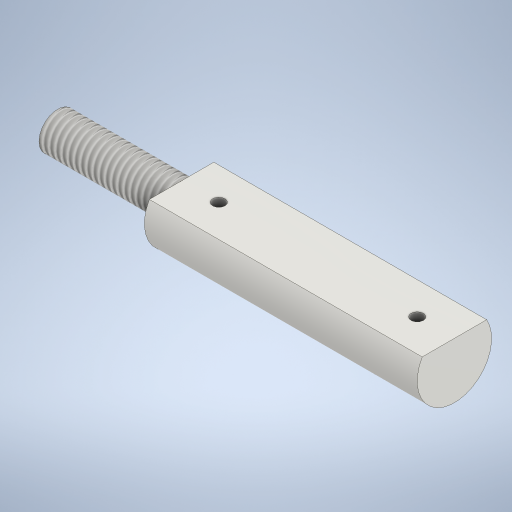
# Autodesk Inventor part: centre shaft
Saved by Autodesk Inventor 2023 (Build 270158000, 158)
## iProperties
CustomPartVersion: 1
Created: 2023-05-29
Part Number: centre shaft
Material: Steel
Document SubType Name: Modeling
Designer: Ronan
Density: 1 g/cm^3
Appearance: Steel
Length: 18,000 mm
Author: Ronan
Autodesk Inventor part; units mm, degrees
ref_plane "Start Plane" through (0, 0, 0) normal (1, 0, 0) x (0, 1, 0)
ref_plane "XZ Plane" through (0, 0, 0) normal (0, 1, 0) x (-1, 0, 0)
ref_plane "XY Plane" through (0, 0, 0) normal (0, 0, 1) x (1, 0, 0)
sketch "Sketch4" plane through (0, 0, 0) normal (1, 0, 0) x (0, 1, 0)
  circle A0 centre (0, 0) radius 3
  dimension "d11" = 6
  constraints: 1 centre point, 1 coincident
  measures "d11" diameter of A0
extrude "Extrusion2" add sketch "Sketch4" along normal blind 22
sketch "Sketch5" plane through (22, 0, 0) normal (1, 0, 0) x (0, 0, -1)
  circle A0 centre (0, 0) radius 3 projected
  line L0 (-2.5981, 1.5) -> (2.5981, 1.5)
  circle A1 centre (0, 0) radius 3
  dimension "d14" = 1.5
  constraints: 2 end point, 2 point on circle, 1 centre point, 1 coincident, 1 concentric, 1 horizontal
  measures "d14" distance from line of point (0, 0) L0
extrude "Extrusion3" cut sketch "Sketch5" against normal through all contours L0 A0 picked at (0.7274, 1.6862)
sketch "Sketch6" plane through (0, 0, 0) normal (-1, 0, 0) x (0, 0, 1)
  circle A0 centre (0, 0) radius 1.5
  dimension "d17" = 3
  constraints: 1 centre point, 1 coincident
  measures "d17" diameter of A0
extrude "Extrusion4" add sketch "Sketch6" along normal blind 10
thread "Thread1" size "M3x0.5" class "6g" standard "ANSI Metric M Profile" full length
sketch "Sketch7" plane through (22, 1.5, 2.5981) normal (0, 1, 0) x (1, 0, 0)
  circle A0 centre (-19, 2.5981) radius 0.5
  circle A1 centre (-3, 2.5981) radius 0.5
  point P0 (-22, 2.5981)
  dimension "d22" = 1
  dimension "d23" = 3
  dimension "d24" = 15
  dimension "d25" = 16
  constraints: 2 centre point, 2 horizontal alignment
  measures "d22" diameter of A0
  measures "d23" distance of A0.centre point (-22, 2.598)
  measures "d25" distance of A0.centre A1.centre
extrude "Extrusion5" cut sketch "Sketch7" against normal through all
equation "\"Length\" = 18"
body "Solid2"
